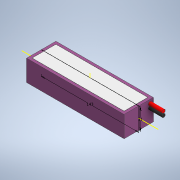
# Autodesk Inventor part: Akku
Saved by Autodesk Inventor 2021 (Build 250183000, 183)
## iProperties
Created: 2020-12-16
Part Number: Akku
Material: Generisch
Document SubType Name: Modeling
Designer: laure
Density: 1 g/cm^3
Appearance: Vorgabe
Author: laure
Autodesk Inventor part; units mm, degrees
ref_plane "YZ Plane" through (0, 0, 0) normal (1, 0, 0) x (0, 1, 0)
ref_plane "XZ Plane" through (0, 0, 0) normal (0, 1, 0) x (-1, 0, 0)
ref_plane "XY Plane" through (0, 0, 0) normal (0, 0, 1) x (1, 0, 0)
sketch "Skizze1" plane through (0, 0, 0) normal (0, 0, 1) x (1, 0, 0)
  line L0 (-71.5, 15.5) -> (71.5, 15.5)
  line L1 (71.5, 15.5) -> (71.5, -15.5)
  line L2 (71.5, -15.5) -> (-71.5, -15.5)
  line L3 (-71.5, -15.5) -> (-71.5, 15.5)
  line L4 (0, -21.7) -> (0, 21.7) projected
  line L5 (-100.1, 0) -> (100.1, 0) projected
  point P0 (0, 0)
  dimension "d0" = 143
  dimension "d1" = 31
  constraints: 8 end point, 2 parallel, 1 horizontal, 1 perpendicular, 2 other
  measures "d0" distance of L1.end L2.end
  measures "d1" distance of L0.end L1.end
extrude "Extrusion1" add sketch "Skizze1" against normal mid plane 43
sketch "Skizze2" plane through (-71.5, 15.5, -21.5) normal (0, 1, 0) x (1, 0, 0)
  line L0 (4, -4) -> (139, -4)
  line L1 (139, -4) -> (139, -39)
  line L2 (139, -39) -> (4, -39)
  line L3 (4, -39) -> (4, -4)
  line L4 (143, -43) -> (0, -43) projected
  line L5 (0, 0) -> (143, 0) projected
  line L6 (0, 0) -> (0, -43) projected
  line L7 (143, 0) -> (143, -43) projected
  point P0 (71.5, -21.5)
  dimension "d5" = 4
  dimension "d6" = 4
  dimension "d7" = 4
  dimension "d8" = 4
  constraints: 8 end point, 2 parallel, 1 horizontal, 1 perpendicular
  measures "d5" distance between parallel lines of L2 L4
  measures "d6" distance between parallel lines of L5 L0
  measures "d7" distance between parallel lines of L6 L3
  measures "d8" distance between parallel lines of L1 L7
extrude "Extrusion2" add sketch "Skizze2" along normal blind 0.2 contours L0 L1 L2 L3
sketch "Skizze3" plane through (71.5, -15.5, -21.5) normal (1, 0, 0) x (0, 0, -1)
  circle A0 centre (-5, 26) radius 2.5
  line L0 (0, 31) -> (-43, 31) projected
  line L1 (0, 31) -> (0, 0) projected
  circle A1 centre (-5, 20.5) radius 2.5
  point P0 (-21.5, 15.5)
  dimension "d11" = 5
  dimension "d12" = 5
  dimension "d13" = 5
  dimension "d14" = 5
  dimension "d15" = 5
  dimension "d16" = 5.5
  constraints: 2 centre point
  measures "d11" diameter of A0
  measures "d12" distance from line of L0 A0.centre
  measures "d13" distance from line of A0.centre L1
  measures "d14" diameter of A1
  measures "d15" distance from line of L1 A1.centre
  measures "d16" distance of A0.centre A1.centre
extrude "Extrusion3" add sketch "Skizze3" along normal blind 20
